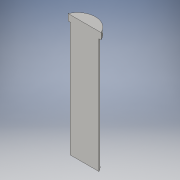
# Autodesk Inventor part: Pin Place holder
Saved by Autodesk Inventor 2016 (Build 200138000, 138)
## iProperties
Created: 2017-03-28
Part Number: Pin Place holder
Material: Generic
Document SubType Name: Modeling
Designer: fmhsr119
Density: 1 g/cm^3
Appearance: Default
Author: fmhsr119
Autodesk Inventor part; units mm, degrees
ref_plane "YZ Plane" through (0, 0, 0) normal (1, 0, 0) x (0, 1, 0)
ref_plane "XZ Plane" through (0, 0, 0) normal (0, 1, 0) x (-1, 0, 0)
ref_plane "XY Plane" through (0, 0, 0) normal (0, 0, 1) x (1, 0, 0)
sketch "Sketch1" plane through (0, 0, 0) normal (0, 1, 0) x (-1, 0, 0)
  circle A0 centre (0, 0) radius 6.35
  dimension "d0" = 12.7
  constraints: 1 centre point, 1 coincident
  measures "d0" diameter of A0
extrude "Extrusion1" add sketch "Sketch1" along normal blind 38.1
sketch "Sketch2" plane through (0, 38.1, 0) normal (0, 1, 0) x (1, 0, 0)
  circle A0 centre (0, 0) radius 7.112
  dimension "d3" = 14.224
  constraints: 1 centre point, 1 coincident
  measures "d3" diameter of A0
extrude "Extrusion2" add sketch "Sketch2" along normal blind 2.54
sketch "Sketch3" plane through (0, 0, 0) normal (0, -1, 0) x (1, 0, 0)
  line L0 (-6.35, -2.794) -> (6.35, -2.794)
  line L1 (6.35, -2.794) -> (6.35, 2.794)
  line L2 (6.35, 2.794) -> (-6.35, 2.794)
  line L3 (-6.35, 2.794) -> (-6.35, -2.794)
  point P0 (0, 0)
  dimension "d6" = 5.588
  constraints: 8 end point, 2 horizontal, 2 parallel, 1 perpendicular
  measures "d6" distance of L2.end L0.start
extrude "Extrusion3" cut sketch "Sketch3" against normal blind 1.27
sketch "Sketch4" plane through (0, 1.27, 0) normal (0, -1, 0) x (1, 0, 0)
  line L0 (5.7023, -2.794) -> (-5.7023, -2.794) projected
  line L1 (5.7023, -2.794) -> (-11.0724, -2.794)
  line L2 (-11.0724, -2.794) -> (-11.0724, 8.6812)
  line L3 (-11.0724, 8.6812) -> (5.7023, 8.6812)
  line L4 (5.7023, 8.6812) -> (5.7023, -2.794)
  line L5 (-11.0724, -2.794) -> (15.5291, -2.794)
  line L6 (15.5291, -2.794) -> (15.5291, 8.6812)
  line L7 (15.5291, 8.6812) -> (-11.0724, 8.6812)
  line L8 (-11.0724, 8.6812) -> (-11.0724, -2.794)
  point P0 (0, 0)
  constraints: 16 end point, 4 parallel, 2 horizontal, 2 perpendicular
sketch "Sketch5" plane through (0, 1.27, 0) normal (0, -1, 0) x (1, 0, 0)
  line L0 (8.174, 2.794) -> (-7.6116, 2.794)
  line L1 (-7.6116, 2.794) -> (-7.6116, -2.794)
  line L2 (-7.6116, -2.794) -> (8.174, -2.794)
  line L3 (8.174, -2.794) -> (8.174, 2.794)
  point P0 (0, 0)
  constraints: 8 end point, 2 parallel, 1 horizontal, 1 perpendicular
extrude "Extrusion4" cut sketch "Sketch5" against normal blind 0.5588
extrude "Extrusion5" cut sketch "Sketch4" against normal up to next
sketch "Sketch6" plane through (0, 0, 0) normal (0, -1, 0) x (1, 0, 0)
  line L0 (14.7281, 0) -> (-10.6227, 0)
  line L1 (-10.6227, 0) -> (-10.6227, 18.3203)
  line L2 (-10.6227, 18.3203) -> (14.7281, 18.3203)
  line L3 (14.7281, 18.3203) -> (14.7281, 0)
  point P0 (0, 0)
  constraints: 8 end point, 2 parallel, 1 horizontal, 1 perpendicular
extrude "Extrusion6" cut sketch "Sketch6" against normal blind 25.4
sketch "Sketch7" plane through (0, 0, 0) normal (0, -1, 0) x (1, 0, 0)
  arc A0 (-5.7023, -2.794) -> (5.7023, -2.794) centre (0, 0) ccw projected
  line L0 (-5.7023, -2.794) -> (-6.5402, -2.794) projected
  line L1 (5.7023, -2.794) -> (-5.7023, -2.794)
  arc A1 (-5.7023, -2.794) -> (5.7023, -2.794) centre (0, 0) ccw
  constraints: 2 end point, 2 point on circle, 1 centre point, 1 horizontal
extrude "Extrusion7" add sketch "Sketch7" along normal blind 7.62
body "Solid1"
